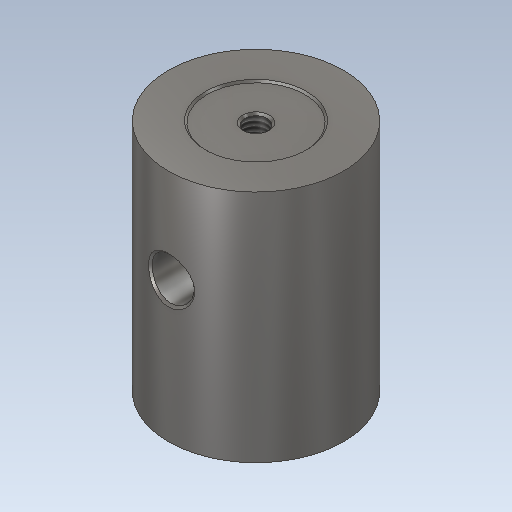
# Autodesk Inventor part: PLS-P642H0335A00_M
Saved by Autodesk Inventor 2020 (Build 240168000, 168)
## iProperties
Created: 2017-06-30
Part Number: PLS-P642H0335A00_M
Material: Stainless Steel
Document SubType Name: Modeling
Designer: map
Density: 8 g/cm^3
Appearance: Semi-Polished
Author: map
Autodesk Inventor part; units mm, degrees
ref_plane "YZ Plane" through (0, 0, 0) normal (1, 0, 0) x (0, 1, 0)
ref_plane "XZ Plane" through (0, 0, 0) normal (0, 1, 0) x (-1, 0, 0)
ref_plane "XY Plane" through (0, 0, 0) normal (0, 0, 1) x (1, 0, 0)
sketch "Sketch1" plane through (0, 0, 0) normal (0, 1, 0) x (-1, 0, 0)
  circle A0 centre (0, 0) radius 12.5
  dimension "d0" = 25
  constraints: 1 centre point, 1 coincident
  measures "d0" diameter of A0
extrude "Extrusion1" add sketch "Sketch1" along normal blind 33.5
hole "ReliefTop" at (0, 33.5, 0) direction (0, -1, 0) diameter 13.97 depth 0.254 countersink diameter 14.478 countersink angle 90
hole "ReliefBottom" at (0, 0, 0) direction (0, 1, 0) diameter 13.97 depth 0.254 countersink diameter 14.478 countersink angle 90
hole "MountBottomM6" at (0, 0.254, 0) direction (0, 1, 0) diameter 4.917 depth 7.366 tip angle 118 countersink diameter 5.508 countersink angle 90 thread size "M6x1" class "6H" standard "ISO Metric profile"
hole "MountTopM4" at (0, 33.246, 0) direction (0, -1, 0) diameter 3.242 depth 14.478 tip angle 118 countersink diameter 3.808 countersink angle 90 thread size "M4x0.7" class "6H" standard "ISO Metric profile"
sketch "Sketch2" plane through (0, 0, 0) normal (0, 0, 1) x (1, 0, 0)
  circle A0 centre (0, 20) radius 3
  line L0 (-12.5, 0) -> (12.5, 0) projected
  line L1 (0, -4.6) -> (0, 27.6) projected
  point P0 (0, 0)
  dimension "d49" = 6
  dimension "d50" = 20
  constraints: 1 centre point, 1 point on line
  measures "d49" diameter of A0
  measures "d50" distance from line of A0.centre L0
extrude "Extrusion2" cut sketch "Sketch2" along normal through all both and the other way through all
chamfer "Chamfer1" distance 0.313 angle 45 2 edges at (-3, 19.9998, 12.1347) (-3, 19.9998, -12.1347)
extrude "Extrusion3" add sketch "Sketch2" along normal mid plane 14.84
equation "\"d1\" = height"
equation "\"d5\" = reliefMinor"
equation "\"d7\" = reliefMajor"
equation "\"d10\" = reliefDepth"
equation "\"d14\" = reliefMinor"
equation "\"d16\" = reliefMajor"
equation "\"d19\" = reliefDepth"
equation "\"d25\" = chamferM6"
equation "\"d28\" = depthM6"
equation "\"d40\" = chamferM4"
equation "\"d43\" = depthM4"
equation "\"reliefDepth\" = 0.254"
equation "\"reliefMinor\" = 13.97"
equation "\"reliefMajor\" = 14.478"
equation "\"chamferM6\" = 5.508"
equation "\"chamferM4\" = 3.808"
equation "\"depthM6\" = 7.366"
equation "\"depthM4\" = 14.478"
equation "\"height\" = 33.5"
body "Solid1"
